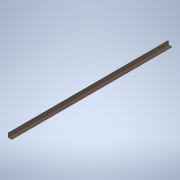
# Autodesk Inventor part: Angulo en V
Saved by Autodesk Inventor 2021 (Build 250183000, 183)
## iProperties
Created: 2021-06-05
Part Number: Angulo en V
Material: Generic
Document SubType Name: Modeling
Designer: Nelson
Density: 1 g/cm^3
Appearance: Default
Author: Nelson
Autodesk Inventor part; units mm, degrees
ref_plane "YZ Plane" through (0, 0, 0) normal (1, 0, 0) x (0, 1, 0)
ref_plane "XZ Plane" through (0, 0, 0) normal (0, 1, 0) x (-1, 0, 0)
ref_plane "XY Plane" through (0, 0, 0) normal (0, 0, 1) x (1, 0, 0)
sketch "Sketch1" plane through (0, 0, 0) normal (0, 0, 1) x (1, 0, 0)
  line L0 (0, 0) -> (0, 30)
  line L1 (0, 0) -> (30, 0)
  line L2 (2, 30) -> (2, 2)
  line L3 (2, 2) -> (30, 2)
  line L4 (0, 30) -> (2, 30)
  line L5 (30, 2) -> (30, 0)
  dimension "d7" = 30
  dimension "d8" = 30
  dimension "d9" = 2
  constraints: 12 end point, 2 horizontal, 1 perpendicular, 1 vertical, 1 other
  measures "d7" distance of L0.start L0.end
  measures "d8" distance of L0.start L1.end
  measures "d9" distance between parallel lines of L0 L2
extrude "Extrusion1" add sketch "Sketch1" against normal blind 1261.8
ref_plane "Work Plane1" through (2, 30, 0) normal (-0.7071068, -0.7071068, 0) x (0, 0, -1)
ref_plane "Work Plane2" through (0, 30, 0) normal (-0.7071068, 0.7071068, 0) x (0, 0, -1)
ref_plane "Work Plane3" through (30, 0, 0) normal (-0.7071068, 0.7071068, 0) x (0, 0, -1)
fillet "Fillet1" radius 2 1 edges at (0, 0, -630.9)
ref_plane "Work Plane4" through (15.0001, 14.9999, 0) normal (-0.7071068, 0.7071068, 0) x (0, 0, -1)
body "Solid1"
